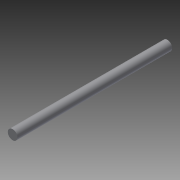
# Autodesk Inventor part: tension_bolt
Saved by Autodesk Inventor 2015 SP1 (Build 190203100, 203)
## iProperties
Created: 2014-12-28
Part Number: tension_bolt
Material: Generic
Document SubType Name: Modeling
Designer: Jarod
Density: 1 g/cm^3
Appearance: Default
Author: Jarod
Autodesk Inventor part; units mm, degrees
ref_plane "YZ Plane" through (0, 0, 0) normal (1, 0, 0) x (0, 1, 0)
ref_plane "XZ Plane" through (0, 0, 0) normal (0, 1, 0) x (-1, 0, 0)
ref_plane "XY Plane" through (0, 0, 0) normal (0, 0, 1) x (1, 0, 0)
sketch "Sketch2" plane through (0, 0, 0) normal (0, 1, 0) x (-1, 0, 0)
  line L0 (0, 0) -> (0, -101.6)
  line L1 (0, 0) -> (101.6, 0) construction
  line L2 (0, -101.6) -> (0, -114.3) construction
  line L3 (-12.7, -127) -> (12.7, -127) construction
  line L4 (12.7, -127) -> (12.7, -101.6) construction
  line L5 (12.7, -101.6) -> (-12.7, -101.6) construction
  line L6 (-12.7, -101.6) -> (-12.7, -127) construction
  line L7 (-12.7, -127) -> (12.7, -101.6) construction
  line L8 (12.7, -127) -> (-12.7, -101.6) construction
  arc A0 (12.7, -114.3) -> (0, -101.6) centre (0, -114.3) ccw
  arc A1 (0, -127) -> (12.7, -114.3) centre (0, -114.3) ccw
  arc A2 (-12.7, -114.3) -> (0, -127) centre (0, -114.3) ccw
  dimension "d3" = 101.6
  dimension "d4" = 90
  dimension "d5" = 12.7
  dimension "d6" = 25.4
  dimension "d7" = 25.4
  dimension "d8" = 12.7
  dimension "d9" = 12.7
  dimension "d10" = 12.7
  constraints: 18 end point, 6 point on circle, 5 midpoint, 3 centre point, 2 horizontal, 2 parallel, 2 perpendicular, 2 vertical
  measures "d3" distance of L0.start L0.end
  measures "d4" angle of L0 L1
  measures "d5" distance of L0.end L2.end
  measures "d6" distance of L5.end L4.end
  measures "d7" distance of L4.end L3.end
  measures "d8" radius of A0
  measures "d9" radius of A1
  measures "d10" radius of A2
sketch "Sketch3" plane through (0, 0, 0) normal (0, 0, 1) x (1, 0, 0)
  circle A0 centre (0, 0) radius 3.175
  dimension "d11" = 6.35
  constraints: 1 centre point, 1 coincident
  measures "d11" diameter of A0
sweep "Sweep1" add profiles "Sketch3" path "Sketch2"
body "Solid2"
